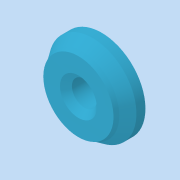
# Autodesk Inventor part: SpurGearThrustDistributer
Saved by Autodesk Inventor 2017 (Build 210142000, 142)
## iProperties
Created: 2016-11-28
Part Number: SpurGearThrustDistributer
Material: ABS Plastic
Document SubType Name: Modeling
Designer: techn
Density: 1.06 g/cm^3
Appearance: Turquoise
Author: techn
Autodesk Inventor part; units mm, degrees
ref_plane "YZ Plane" through (0, 0, 0) normal (1, 0, 0) x (0, 1, 0)
ref_plane "XZ Plane" through (0, 0, 0) normal (0, 1, 0) x (-1, 0, 0)
ref_plane "XY Plane" through (0, 0, 0) normal (0, 0, 1) x (1, 0, 0)
sketch "Sketch2" plane through (0, 0, 0) normal (0, 0, 1) x (1, 0, 0)
  circle A0 centre (0, 0) radius 4.5085
  circle A1 centre (0, 0) radius 15.875
  dimension "d3" = 9.017
  dimension "d4" = 31.75
  constraints: 2 centre point, 2 coincident
  measures "d3" diameter of A0
  measures "d4" diameter of A1
extrude "Extrusion2" add sketch "Sketch2" along normal blind 8.382
chamfer "Chamfer1" distance 2.159 angle 45 1 edges at (-4.5085, 0, 8.382)
sketch "Sketch6" plane through (0, 0, 0) normal (0, 1, 0) x (-1, 0, 0)
  line L0 (15.875, 8.382) -> (-15.875, 8.382) projected
  line L1 (-15.875, 0) -> (15.875, 0) projected
  line L2 (15.875, 8.382) -> (12.7, 8.382)
  line L3 (15.875, 8.382) -> (-15.875, 8.382) projected
  line L4 (15.875, 8.382) -> (15.875, 6.9533)
  line L5 (15.875, 0) -> (15.875, 8.382) projected
  line L6 (15.875, 6.9533) -> (13.335, 6.9533)
  line L7 (13.335, 6.9533) -> (12.7, 8.382)
  line L8 (0, 0) -> (0, 8.967)
  dimension "d21" = 3.175
  dimension "d22" = 1.4287
  dimension "d23" = 2.54
  constraints: 10 end point, 2 point on line, 1 perpendicular, 1 vertical
  measures "d21" distance of L0.start L2.end
  measures "d22" distance of L0.start L4.end
  measures "d23" distance of L4.end L6.end
revolve "Revolution1" cut sketch "Sketch6" angle 360 about axis through (0, 0, 0) along (0, 0, 1) contours L4 L6 L7 L0
sketch "Sketch7" plane through (0, 0, 0) normal (0, 0, -1) x (-1, 0, 0)
  line L0 (-3.3729, 8.3312) -> (-1.6864, 11.2522)
  line L1 (-1.6864, 11.2522) -> (1.6864, 11.2522)
  line L2 (1.6864, 11.2522) -> (3.3729, 8.3312)
  line L3 (3.3729, 8.3312) -> (1.6864, 5.4102)
  line L4 (1.6864, 5.4102) -> (-1.6864, 5.4102)
  line L5 (-1.6864, 5.4102) -> (-3.3729, 8.3312)
  point P0 (0, 0)
  point P1 (0, 8.3312)
  dimension "d27" = 8.3312
  dimension "d28" = 5.842
  constraints: 12 end point, 1 horizontal, 1 vertical alignment, 13 other
  measures "d27" distance of point (0, 0) point (0, 8.331)
  measures "d28" distance between parallel lines of L1 L4
extrude "Extrusion4" cut sketch "Sketch7" against normal blind 4.064
chamfer "Chamfer3" distance 1.27 angle 45 6 edges at (2.5297, 9.7917, 4.064) (0, 11.2522, 4.064) (-2.5297, 9.7917, 4.064) (-2.5297, 6.8707, 4.064) (0, 5.4102, 4.064) (2.5297, 6.8707, 4.064)
pattern_circular "Circular Pattern1" count 3 over 360 about axis through (0, 0, 0) along (0, 0, 1) of "Extrusion4", "Chamfer3"
chamfer "Chamfer4" distance 3.683 distance2 2.54 1 edges at (-15.875, 0, 6.9533) measured on face at (-15.875, 0, 6.4533)
body "Solid2"
